Autodesk Fusion 360 part; units mm, degrees
note: some values were not read from the file. Set by a fixed rule: which sketch regions a step uses.
(part 10 of 20)
  spline S54 degree 5 poles (26.1461, -12.6495) (26.1462, -12.6495) (26.1464, -12.6496) (26.1467, -12.6497) (26.1471, -12.65) (26.1478, -12.6503) (26.1486, -12.6506) (26.1495, -12.651) (26.1504, -12.6515) (26.1515, -12.652) (26.1527, -12.6526) (26.154, -12.6531) (26.1554, -12.6538) (26.1569, -12.6544) (26.1585, -12.6551) (26.1602, -12.6559) (26.1619, -12.6567) (26.1638, -12.6575) (26.1658, -12.6583) (26.1678, -12.6592) (26.17, -12.6602) (26.1722, -12.6611) (26.1745, -12.6621) (26.1769, -12.6631) (26.1794, -12.6642) (26.182, -12.6653) (26.1847, -12.6664) (26.1874, -12.6676) (26.1903, -12.6687) (26.1932, -12.6699) (26.1962, -12.6712) (26.1993, -12.6724) (26.2024, -12.6737) (26.2057, -12.675) (26.209, -12.6764) (26.2124, -12.6778) (26.2159, -12.6791) (26.2195, -12.6806) (26.2231, -12.682) (26.2269, -12.6834) (26.2307, -12.6849) (26.2345, -12.6864) (26.2385, -12.688) (26.2425, -12.6895) (26.2466, -12.6911) (26.2508, -12.6927) (26.255, -12.6943) (26.2594, -12.6959) (26.2638, -12.6975) (26.2682, -12.6992) (26.2728, -12.7009) (26.2774, -12.7026) (26.282, -12.7043) (26.2868, -12.706) (26.2916, -12.7077) (26.2965, -12.7095) (26.3015, -12.7113) (26.3065, -12.7131) (26.3116, -12.7149) (26.3167, -12.7167) (26.322, -12.7185) (26.3273, -12.7204) (26.3326, -12.7222) (26.338, -12.7241) (26.3435, -12.726) (26.3491, -12.7279) (26.3547, -12.7298) (26.3604, -12.7317) (26.3661, -12.7336) (26.3719, -12.7356) (26.3778, -12.7375) (26.3837, -12.7395) (26.3897, -12.7414) (26.3958, -12.7434) (26.4019, -12.7454) (26.4081, -12.7474) (26.4144, -12.7494) (26.4207, -12.7514) (26.427, -12.7534) (26.4335, -12.7555) (26.4399, -12.7575) (26.4465, -12.7596) (26.4531, -12.7616) (26.4598, -12.7637) (26.4665, -12.7657) (26.4733, -12.7678) (26.4801, -12.7699) (26.487, -12.772) (26.4939, -12.774) (26.5009, -12.7761) (26.508, -12.7782) (26.5151, -12.7803) (26.5223, -12.7824) (26.5296, -12.7845) (26.5368, -12.7867) (26.5442, -12.7888) (26.5516, -12.7909) (26.559, -12.793) (26.5665, -12.7952) (26.5741, -12.7973) (26.5817, -12.7994) (26.5894, -12.8016) (26.5971, -12.8037) (26.6049, -12.8058) (26.6127, -12.808) (26.6206, -12.8101) (26.6286, -12.8123) (26.6365, -12.8144) (26.6446, -12.8166) (26.6527, -12.8187) (26.6608, -12.8208) (26.669, -12.823) (26.6773, -12.8251) (26.6856, -12.8273) (26.6939, -12.8294) (26.7023, -12.8316) (26.7108, -12.8337) (26.7193, -12.8359) (26.7278, -12.838) (26.7364, -12.8402) (26.7451, -12.8423) (26.7537, -12.8445) (26.7625, -12.8466) (26.7713, -12.8487) (26.7801, -12.8509) (26.789, -12.853) (26.798, -12.8551) (26.8069, -12.8573) (26.816, -12.8594) (26.8251, -12.8615) (26.8342, -12.8636) (26.8434, -12.8658) (26.8526, -12.8679) (26.8619, -12.87) (26.8712, -12.8721) (26.8806, -12.8742) (26.89, -12.8763) (26.8994, -12.8784) (26.9089, -12.8805) (26.9185, -12.8826) (26.9281, -12.8847) (26.9377, -12.8867) (26.9474, -12.8888) (26.9571, -12.8909) (26.9669, -12.8929) (26.9767, -12.895) (26.9866, -12.8971) (26.9965, -12.8991) (27.0064, -12.9011) (27.0164, -12.9032) (27.0265, -12.9052) (27.0365, -12.9072) (27.0467, -12.9093) (27.0568, -12.9113) (27.0671, -12.9133) (27.0773, -12.9153) (27.0876, -12.9173) (27.0979, -12.9193) (27.1083, -12.9213) (27.1188, -12.9232) (27.1292, -12.9252) (27.1397, -12.9272) (27.1503, -12.9291) (27.1609, -12.9311) (27.1715, -12.933) (27.1822, -12.9349) (27.1929, -12.9368) (27.2037, -12.9388) (27.2145, -12.9407) (27.2253, -12.9426) (27.2362, -12.9445) (27.2471, -12.9463) (27.2581, -12.9482) (27.2691, -12.9501) (27.2801, -12.9519) (27.2912, -12.9538) (27.3023, -12.9556) (27.3135, -12.9574) (27.3247, -12.9593) (27.3359, -12.9611) (27.3472, -12.9629) (27.3585, -12.9647) (27.3699, -12.9665) (27.3813, -12.9682) (27.3927, -12.97) (27.4042, -12.9718) (27.4157, -12.9735) (27.4273, -12.9752) (27.4388, -12.977) (27.4505, -12.9787) (27.4621, -12.9804) (27.4738, -12.9821) (27.4856, -12.9838) (27.4974, -12.9854) (27.5092, -12.9871) (27.521, -12.9887) (27.5329, -12.9904) (27.5449, -12.992) (27.5568, -12.9936) (27.5688, -12.9952) (27.5809, -12.9968) (27.5929, -12.9984) (27.605, -13) (27.6172, -13.0016) (27.6294, -13.0031) (27.6416, -13.0047) (27.6539, -13.0062) (27.6661, -13.0077) (27.6785, -13.0092) (27.6908, -13.0107) (27.7032, -13.0122) (27.7157, -13.0136) (27.7281, -13.0151) (27.7406, -13.0165) (27.7532, -13.018) (27.7658, -13.0194) (27.7784, -13.0208) (27.791, -13.0222) (27.8037, -13.0236) (27.8164, -13.0249) (27.8291, -13.0263) (27.8419, -13.0276) (27.8547, -13.029) (27.8676, -13.0303) (27.8805, -13.0316) (27.8934, -13.0329) (27.9063, -13.0342) (27.9193, -13.0354) (27.9323, -13.0367) (27.9454, -13.0379) (27.9585, -13.0391) (27.9716, -13.0404) (27.9848, -13.0415) (27.9979, -13.0427) (28.0112, -13.0439) (28.0244, -13.0451) (28.0377, -13.0462) (28.051, -13.0473) (28.0644, -13.0484) (28.0777, -13.0495) (28.0911, -13.0506) (28.1019, -13.0515) (28.11, -13.0521) (28.1154, -13.0525) (28.1181, -13.0527) knots 0 0 0 0 0 0 0.00416667 0.00833333 0.0125 0.01666667 0.02083333 0.025 0.02916667 0.03333333 0.0375 0.04166667 0.04583333 0.05 0.05416667 0.05833333 0.0625 0.06666667 0.07083333 0.075 0.07916667 0.08333333 0.0875 0.09166667 0.09583333 0.1 0.10416667 0.10833333 0.1125 0.11666667 0.12083333 0.125 0.12916667 0.13333333 0.1375 0.14166667 0.14583333 0.15 0.15416667 0.15833333 0.1625 0.16666667 0.17083333 0.175 0.17916667 0.18333333 0.1875 0.19166667 0.19583333 0.2 0.20416667 0.20833333 0.2125 0.21666667 0.22083333 0.225 0.22916667 0.23333333 0.2375 0.24166667 0.24583333 0.25 0.25416667 0.25833333 0.2625 0.26666667 0.27083333 0.275 0.27916667 0.28333333 0.2875 0.29166667 0.29583333 0.3 0.30416667 0.30833333 0.3125 0.31666667 0.32083333 0.325 0.32916667 0.33333333 0.3375 0.34166667 0.34583333 0.35 0.35416667 0.35833333 0.3625 0.36666667 0.37083333 0.375 0.37916667 0.38333333 0.3875 0.39166667 0.39583333 0.4 0.40416667 0.40833333 0.4125 0.41666667 0.42083333 0.425 0.42916667 0.43333333 0.4375 0.44166667 0.44583333 0.45 0.45416667 0.45833333 0.4625 0.46666667 0.47083333 0.475 0.47916667 0.48333333 0.4875 0.49166667 0.49583333 0.5 0.50416667 0.50833333 0.5125 0.51666667 0.52083333 0.525 0.52916667 0.53333333 0.5375 0.54166667 0.54583333 0.55 0.55416667 0.55833333 0.5625 0.56666667 0.57083333 0.575 0.57916667 0.58333333 0.5875 0.59166667 0.59583333 0.6 0.60416667 0.60833333 0.6125 0.61666667 0.62083333 0.625 0.62916667 0.63333333 0.6375 0.64166667 0.64583333 0.65 0.65416667 0.65833333 0.6625 0.66666667 0.67083333 0.675 0.67916667 0.68333333 0.6875 0.69166667 0.69583333 0.7 0.70416667 0.70833333 0.7125 0.71666667 0.72083333 0.725 0.72916667 0.73333333 0.7375 0.74166667 0.74583333 0.75 0.75416667 0.75833333 0.7625 0.76666667 0.77083333 0.775 0.77916667 0.78333333 0.7875 0.79166667 0.79583333 0.8 0.80416667 0.80833333 0.8125 0.81666667 0.82083333 0.825 0.82916667 0.83333333 0.8375 0.84166667 0.84583333 0.85 0.85416667 0.85833333 0.8625 0.86666667 0.87083333 0.875 0.87916667 0.88333333 0.8875 0.89166667 0.89583333 0.9 0.90416667 0.90833333 0.9125 0.91666667 0.92083333 0.925 0.92916667 0.93333333 0.9375 0.94166667 0.94583333 0.95 0.95416667 0.95833333 0.9625 0.96666667 0.97083333 0.975 0.97916667 0.98333333 0.9875 0.99166667 0.99583333 1 1 1 1 1 1
  spline S55 degree 5 poles (-25.6019, -13.7175) (-25.602, -13.7175) (-25.6022, -13.7176) (-25.6025, -13.7178) (-25.6029, -13.718) (-25.6036, -13.7184) (-25.6043, -13.7188) (-25.6052, -13.7193) (-25.6061, -13.7198) (-25.6072, -13.7204) (-25.6083, -13.721) (-25.6096, -13.7217) (-25.6109, -13.7225) (-25.6123, -13.7233) (-25.6138, -13.7242) (-25.6154, -13.7251) (-25.6171, -13.7261) (-25.6188, -13.7271) (-25.6207, -13.7282) (-25.6226, -13.7293) (-25.6246, -13.7305) (-25.6267, -13.7317) (-25.6289, -13.733) (-25.6311, -13.7344) (-25.6334, -13.7358) (-25.6358, -13.7372) (-25.6383, -13.7387) (-25.6409, -13.7403) (-25.6435, -13.7419) (-25.6462, -13.7435) (-25.6489, -13.7452) (-25.6518, -13.747) (-25.6547, -13.7488) (-25.6577, -13.7506) (-25.6607, -13.7526) (-25.6638, -13.7545) (-25.667, -13.7565) (-25.6702, -13.7586) (-25.6735, -13.7607) (-25.6769, -13.7628) (-25.6803, -13.765) (-25.6838, -13.7673) (-25.6874, -13.7696) (-25.691, -13.7719) (-25.6947, -13.7743) (-25.6984, -13.7768) (-25.7022, -13.7793) (-25.706, -13.7818) (-25.71, -13.7844) (-25.7139, -13.787) (-25.718, -13.7897) (-25.722, -13.7925) (-25.7262, -13.7952) (-25.7304, -13.7981) (-25.7346, -13.8009) (-25.7389, -13.8039) (-25.7432, -13.8068) (-25.7476, -13.8098) (-25.7521, -13.8129) (-25.7566, -13.816) (-25.7612, -13.8192) (-25.7658, -13.8224) (-25.7704, -13.8256) (-25.7751, -13.8289) (-25.7799, -13.8322) (-25.7847, -13.8356) (-25.7895, -13.839) (-25.7944, -13.8425) (-25.7993, -13.846) (-25.8043, -13.8496) (-25.8093, -13.8532) (-25.8144, -13.8568) (-25.8195, -13.8605) (-25.8247, -13.8643) (-25.8299, -13.8681) (-25.8352, -13.8719) (-25.8405, -13.8758) (-25.8458, -13.8797) (-25.8512, -13.8836) (-25.8566, -13.8876) (-25.8621, -13.8917) (-25.8676, -13.8958) (-25.8731, -13.8999) (-25.8787, -13.9041) (-25.8843, -13.9083) (-25.89, -13.9126) (-25.8957, -13.9169) (-25.9014, -13.9213) (-25.9072, -13.9257) (-25.913, -13.9301) (-25.9188, -13.9346) (-25.9247, -13.9391) (-25.9306, -13.9437) (-25.9366, -13.9483) (-25.9426, -13.9529) (-25.9486, -13.9576) (-25.9547, -13.9624) (-25.9608, -13.9672) (-25.9669, -13.972) (-25.9731, -13.9769) (-25.9793, -13.9818) (-25.9855, -13.9867) (-25.9918, -13.9917) (-25.9981, -13.9967) (-26.0044, -14.0018) (-26.0108, -14.0069) (-26.0172, -14.0121) (-26.0236, -14.0173) (-26.0301, -14.0225) (-26.0366, -14.0278) (-26.0431, -14.0332) (-26.0497, -14.0385) (-26.0563, -14.0439) (-26.0629, -14.0494) (-26.0695, -14.0549) (-26.0762, -14.0604) (-26.0829, -14.066) (-26.0896, -14.0716) (-26.0964, -14.0772) (-26.1032, -14.0829) (-26.11, -14.0887) (-26.1168, -14.0945) (-26.1237, -14.1003) (-26.1306, -14.1061) (-26.1375, -14.112) (-26.1445, -14.118) (-26.1515, -14.1239) (-26.1585, -14.13) (-26.1655, -14.136) (-26.1726, -14.1421) (-26.1796, -14.1483) (-26.1868, -14.1544) (-26.1939, -14.1607) (-26.201, -14.1669) (-26.2082, -14.1732) (-26.2154, -14.1796) (-26.2227, -14.1859) (-26.2299, -14.1924) (-26.2372, -14.1988) (-26.2445, -14.2053) (-26.2518, -14.2119) (-26.2592, -14.2184) (-26.2665, -14.225) (-26.2739, -14.2317) (-26.2813, -14.2384) (-26.2888, -14.2451) (-26.2962, -14.2519) (-26.3037, -14.2587) (-26.3112, -14.2656) (-26.3188, -14.2724) (-26.3263, -14.2794) (-26.3339, -14.2863) (-26.3414, -14.2933) (-26.3491, -14.3004) (-26.3567, -14.3075) (-26.3643, -14.3146) (-26.372, -14.3217) (-26.3797, -14.3289) (-26.3874, -14.3362) (-26.3951, -14.3435) (-26.4029, -14.3508) (-26.4106, -14.3581) (-26.4184, -14.3655) (-26.4262, -14.3729) (-26.434, -14.3804) (-26.4419, -14.3879) (-26.4497, -14.3954) (-26.4576, -14.403) (-26.4655, -14.4106) (-26.4734, -14.4183) (-26.4813, -14.426) (-26.4893, -14.4337) (-26.4972, -14.4415) (-26.5052, -14.4493) (-26.5132, -14.4571) (-26.5212, -14.465) (-26.5292, -14.4729) (-26.5373, -14.4809) (-26.5453, -14.4889) (-26.5534, -14.4969) (-26.5615, -14.505) (-26.5696, -14.5131) (-26.5777, -14.5212) (-26.5858, -14.5294) (-26.594, -14.5376) (-26.6022, -14.5459) (-26.6103, -14.5541) (-26.6185, -14.5625) (-26.6267, -14.5708) (-26.635, -14.5792) (-26.6432, -14.5877) (-26.6514, -14.5961) (-26.6597, -14.6046) (-26.668, -14.6132) (-26.6763, -14.6218) (-26.6846, -14.6304) (-26.6929, -14.639) (-26.7012, -14.6477) (-26.7096, -14.6565) (-26.7179, -14.6652) (-26.7263, -14.674) (-26.7347, -14.6829) (-26.7431, -14.6917) (-26.7515, -14.7006) (-26.7599, -14.7096) (-26.7683, -14.7186) (-26.7767, -14.7276) (-26.7852, -14.7366) (-26.7937, -14.7457) (-26.8021, -14.7549) (-26.8106, -14.764) (-26.8191, -14.7732) (-26.8276, -14.7824) (-26.8361, -14.7917) (-26.8447, -14.801) (-26.8532, -14.8104) (-26.8618, -14.8197) (-26.8703, -14.8291) (-26.8789, -14.8386) (-26.8875, -14.8481) (-26.8961, -14.8576) (-26.9047, -14.8671) (-26.9133, -14.8767) (-26.9219, -14.8863) (-26.9305, -14.896) (-26.9392, -14.9057) (-26.9478, -14.9154) (-26.9565, -14.9252) (-26.9651, -14.935) (-26.9738, -14.9448) (-26.9825, -14.9547) (-26.9912, -14.9646) (-26.9999, -14.9745) (-27.0086, -14.9845) (-27.0173, -14.9945) (-27.026, -15.0045) (-27.0347, -15.0146) (-27.0435, -15.0247) (-27.0522, -15.0349) (-27.061, -15.045) (-27.0697, -15.0553) (-27.0767, -15.0635) (-27.082, -15.0696) (-27.0855, -15.0737) (-27.0873, -15.0758) knots 0 0 0 0 0 0 0.00416667 0.00833333 0.0125 0.01666667 0.02083333 0.025 0.02916667 0.03333333 0.0375 0.04166667 0.04583333 0.05 0.05416667 0.05833333 0.0625 0.06666667 0.07083333 0.075 0.07916667 0.08333333 0.0875 0.09166667 0.09583333 0.1 0.10416667 0.10833333 0.1125 0.11666667 0.12083333 0.125 0.12916667 0.13333333 0.1375 0.14166667 0.14583333 0.15 0.15416667 0.15833333 0.1625 0.16666667 0.17083333 0.175 0.17916667 0.18333333 0.1875 0.19166667 0.19583333 0.2 0.20416667 0.20833333 0.2125 0.21666667 0.22083333 0.225 0.22916667 0.23333333 0.2375 0.24166667 0.24583333 0.25 0.25416667 0.25833333 0.2625 0.26666667 0.27083333 0.275 0.27916667 0.28333333 0.2875 0.29166667 0.29583333 0.3 0.30416667 0.30833333 0.3125 0.31666667 0.32083333 0.325 0.32916667 0.33333333 0.3375 0.34166667 0.34583333 0.35 0.35416667 0.35833333 0.3625 0.36666667 0.37083333 0.375 0.37916667 0.38333333 0.3875 0.39166667 0.39583333 0.4 0.40416667 0.40833333 0.4125 0.41666667 0.42083333 0.425 0.42916667 0.43333333 0.4375 0.44166667 0.44583333 0.45 0.45416667 0.45833333 0.4625 0.46666667 0.47083333 0.475 0.47916667 0.48333333 0.4875 0.49166667 0.49583333 0.5 0.50416667 0.50833333 0.5125 0.51666667 0.52083333 0.525 0.52916667 0.53333333 0.5375 0.54166667 0.54583333 0.55 0.55416667 0.55833333 0.5625 0.56666667 0.57083333 0.575 0.57916667 0.58333333 0.5875 0.59166667 0.59583333 0.6 0.60416667 0.60833333 0.6125 0.61666667 0.62083333 0.625 0.62916667 0.63333333 0.6375 0.64166667 0.64583333 0.65 0.65416667 0.65833333 0.6625 0.66666667 0.67083333 0.675 0.67916667 0.68333333 0.6875 0.69166667 0.69583333 0.7 0.70416667 0.70833333 0.7125 0.71666667 0.72083333 0.725 0.72916667 0.73333333 0.7375 0.74166667 0.74583333 0.75 0.75416667 0.75833333 0.7625 0.76666667 0.77083333 0.775 0.77916667 0.78333333 0.7875 0.79166667 0.79583333 0.8 0.80416667 0.80833333 0.8125 0.81666667 0.82083333 0.825 0.82916667 0.83333333 0.8375 0.84166667 0.84583333 0.85 0.85416667 0.85833333 0.8625 0.86666667 0.87083333 0.875 0.87916667 0.88333333 0.8875 0.89166667 0.89583333 0.9 0.90416667 0.90833333 0.9125 0.91666667 0.92083333 0.925 0.92916667 0.93333333 0.9375 0.94166667 0.94583333 0.95 0.95416667 0.95833333 0.9625 0.96666667 0.97083333 0.975 0.97916667 0.98333333 0.9875 0.99166667 0.99583333 1 1 1 1 1 1
  arc A56 (28.1181, -13.0527) -> (28.5147, -12.1618) centre (0, 0) ccw
  line L110 (26.8948, -10.9659) -> (26.6221, -10.8547)
  line L111 (22.1904, -18.7406) -> (22.1898, -18.7401)
  line L112 (-28.2039, -6.9368) -> (-27.918, -6.8665)
  spline S56 degree 5 poles (17.8091, 22.9448) (17.8092, 22.9448) (17.8093, 22.945) (17.8095, 22.9453) (17.8098, 22.9457) (17.8103, 22.9463) (17.8108, 22.9469) (17.8114, 22.9477) (17.812, 22.9486) (17.8127, 22.9496) (17.8135, 22.9506) (17.8144, 22.9518) (17.8153, 22.953) (17.8162, 22.9543) (17.8172, 22.9557) (17.8183, 22.9572) (17.8195, 22.9588) (17.8207, 22.9604) (17.8219, 22.9622) (17.8232, 22.964) (17.8246, 22.9659) (17.826, 22.9679) (17.8274, 22.9699) (17.8289, 22.9721) (17.8305, 22.9743) (17.8321, 22.9766) (17.8337, 22.979) (17.8354, 22.9814) (17.8372, 22.984) (17.8389, 22.9866) (17.8408, 22.9893) (17.8427, 22.992) (17.8446, 22.9948) (17.8465, 22.9978) (17.8485, 23.0007) (17.8506, 23.0038) (17.8527, 23.0069) (17.8548, 23.0101) (17.857, 23.0134) (17.8592, 23.0167) (17.8614, 23.0201) (17.8637, 23.0236) (17.866, 23.0271) (17.8683, 23.0308) (17.8707, 23.0344) (17.8731, 23.0382) (17.8756, 23.042) (17.8781, 23.0459) (17.8806, 23.0499) (17.8831, 23.0539) (17.8857, 23.058) (17.8883, 23.0621) (17.891, 23.0664) (17.8937, 23.0706) (17.8964, 23.075) (17.8991, 23.0794) (17.9019, 23.0839) (17.9047, 23.0884) (17.9075, 23.093) (17.9103, 23.0977) (17.9132, 23.1024) (17.9161, 23.1072) (17.9191, 23.1121) (17.922, 23.117) (17.925, 23.122) (17.928, 23.127) (17.931, 23.1321) (17.9341, 23.1373) (17.9372, 23.1425) (17.9403, 23.1478) (17.9434, 23.1531) (17.9466, 23.1585) (17.9497, 23.164) (17.9529, 23.1695) (17.9562, 23.1751) (17.9594, 23.1807) (17.9627, 23.1864) (17.9659, 23.1921) (17.9692, 23.1979) (17.9726, 23.2038) (17.9759, 23.2097) (17.9793, 23.2157) (17.9826, 23.2217) (17.986, 23.2278) (17.9895, 23.234) (17.9929, 23.2402) (17.9963, 23.2464) (17.9998, 23.2527) (18.0033, 23.2591) (18.0068, 23.2655) (18.0103, 23.272) (18.0139, 23.2785) (18.0174, 23.2851) (18.021, 23.2918) (18.0246, 23.2984) (18.0282, 23.3052) (18.0318, 23.312) (18.0354, 23.3188) (18.039, 23.3257) (18.0427, 23.3327) (18.0464, 23.3397) (18.0501, 23.3468) (18.0538, 23.3539) (18.0575, 23.361) (18.0612, 23.3683) (18.0649, 23.3755) (18.0687, 23.3828) (18.0724, 23.3902) (18.0762, 23.3976) (18.08, 23.4051) (18.0838, 23.4126) (18.0876, 23.4202) (18.0914, 23.4278) (18.0952, 23.4355) (18.0991, 23.4432) (18.1029, 23.451) (18.1068, 23.4588) (18.1106, 23.4666) (18.1145, 23.4746) (18.1184, 23.4825) (18.1223, 23.4905) (18.1262, 23.4986) (18.1301, 23.5067) (18.134, 23.5149) (18.1379, 23.5231) (18.1419, 23.5313) (18.1458, 23.5396) (18.1498, 23.548) (18.1537, 23.5564) (18.1577, 23.5648) (18.1617, 23.5733) (18.1657, 23.5818) (18.1696, 23.5904) (18.1736, 23.5991) (18.1776, 23.6077) (18.1816, 23.6165) (18.1857, 23.6252) (18.1897, 23.634) (18.1937, 23.6429) (18.1977, 23.6518) (18.2018, 23.6607) (18.2058, 23.6697) (18.2098, 23.6788) (18.2139, 23.6879) (18.2179, 23.697) (18.222, 23.7062) (18.226, 23.7154) (18.2301, 23.7247) (18.2342, 23.734) (18.2383, 23.7433) (18.2423, 23.7527) (18.2464, 23.7622) (18.2505, 23.7716) (18.2546, 23.7812) (18.2587, 23.7907) (18.2627, 23.8004) (18.2668, 23.81) (18.2709, 23.8197) (18.275, 23.8295) (18.2791, 23.8393) (18.2832, 23.8491) (18.2873, 23.859) (18.2914, 23.8689) (18.2955, 23.8788) (18.2996, 23.8888) (18.3038, 23.8989) (18.3079, 23.909) (18.312, 23.9191) (18.3161, 23.9292) (18.3202, 23.9395) (18.3243, 23.9497) (18.3284, 23.96) (18.3325, 23.9703) (18.3366, 23.9807) (18.3408, 23.9911) (18.3449, 24.0016) (18.349, 24.0121) (18.3531, 24.0226) (18.3572, 24.0332) (18.3613, 24.0438) (18.3654, 24.0545) (18.3695, 24.0652) (18.3736, 24.0759) (18.3777, 24.0867) (18.3818, 24.0975) (18.3859, 24.1084) (18.39, 24.1193) (18.3941, 24.1302) (18.3982, 24.1412) (18.4023, 24.1522) (18.4064, 24.1633) (18.4105, 24.1744) (18.4146, 24.1855) (18.4187, 24.1967) (18.4228, 24.2079) (18.4269, 24.2191) (18.4309, 24.2304) (18.435, 24.2417) (18.4391, 24.2531) (18.4431, 24.2645) (18.4472, 24.276) (18.4513, 24.2874) (18.4553, 24.299) (18.4594, 24.3105) (18.4634, 24.3221) (18.4675, 24.3337) (18.4715, 24.3454) (18.4756, 24.3571) (18.4796, 24.3689) (18.4836, 24.3806) (18.4877, 24.3925) (18.4917, 24.4043) (18.4957, 24.4162) (18.4997, 24.4281) (18.5037, 24.4401) (18.5077, 24.4521) (18.5117, 24.4642) (18.5157, 24.4762) (18.5197, 24.4884) (18.5237, 24.5005) (18.5277, 24.5127) (18.5316, 24.5249) (18.5356, 24.5372) (18.5395, 24.5495) (18.5435, 24.5618) (18.5475, 24.5742) (18.5514, 24.5866) (18.5553, 24.599) (18.5593, 24.6115) (18.5632, 24.624) (18.5671, 24.6365) (18.571, 24.6491) (18.5749, 24.6617) (18.5788, 24.6744) (18.5827, 24.6871) (18.5866, 24.6998) (18.5905, 24.7125) (18.5943, 24.7253) (18.5982, 24.7382) (18.6021, 24.751) (18.6059, 24.7639) (18.609, 24.7743) (18.6113, 24.782) (18.6128, 24.7872) (18.6136, 24.7898) knots 0 0 0 0 0 0 0.00416667 0.00833333 0.0125 0.01666667 0.02083333 0.025 0.02916667 0.03333333 0.0375 0.04166667 0.04583333 0.05 0.05416667 0.05833333 0.0625 0.06666667 0.07083333 0.075 0.07916667 0.08333333 0.0875 0.09166667 0.09583333 0.1 0.10416667 0.10833333 0.1125 0.11666667 0.12083333 0.125 0.12916667 0.13333333 0.1375 0.14166667 0.14583333 0.15 0.15416667 0.15833333 0.1625 0.16666667 0.17083333 0.175 0.17916667 0.18333333 0.1875 0.19166667 0.19583333 0.2 0.20416667 0.20833333 0.2125 0.21666667 0.22083333 0.225 0.22916667 0.23333333 0.2375 0.24166667 0.24583333 0.25 0.25416667 0.25833333 0.2625 0.26666667 0.27083333 0.275 0.27916667 0.28333333 0.2875 0.29166667 0.29583333 0.3 0.30416667 0.30833333 0.3125 0.31666667 0.32083333 0.325 0.32916667 0.33333333 0.3375 0.34166667 0.34583333 0.35 0.35416667 0.35833333 0.3625 0.36666667 0.37083333 0.375 0.37916667 0.38333333 0.3875 0.39166667 0.39583333 0.4 0.40416667 0.40833333 0.4125 0.41666667 0.42083333 0.425 0.42916667 0.43333333 0.4375 0.44166667 0.44583333 0.45 0.45416667 0.45833333 0.4625 0.46666667 0.47083333 0.475 0.47916667 0.48333333 0.4875 0.49166667 0.49583333 0.5 0.50416667 0.50833333 0.5125 0.51666667 0.52083333 0.525 0.52916667 0.53333333 0.5375 0.54166667 0.54583333 0.55 0.55416667 0.55833333 0.5625 0.56666667 0.57083333 0.575 0.57916667 0.58333333 0.5875 0.59166667 0.59583333 0.6 0.60416667 0.60833333 0.6125 0.61666667 0.62083333 0.625 0.62916667 0.63333333 0.6375 0.64166667 0.64583333 0.65 0.65416667 0.65833333 0.6625 0.66666667 0.67083333 0.675 0.67916667 0.68333333 0.6875 0.69166667 0.69583333 0.7 0.70416667 0.70833333 0.7125 0.71666667 0.72083333 0.725 0.72916667 0.73333333 0.7375 0.74166667 0.74583333 0.75 0.75416667 0.75833333 0.7625 0.76666667 0.77083333 0.775 0.77916667 0.78333333 0.7875 0.79166667 0.79583333 0.8 0.80416667 0.80833333 0.8125 0.81666667 0.82083333 0.825 0.82916667 0.83333333 0.8375 0.84166667 0.84583333 0.85 0.85416667 0.85833333 0.8625 0.86666667 0.87083333 0.875 0.87916667 0.88333333 0.8875 0.89166667 0.89583333 0.9 0.90416667 0.90833333 0.9125 0.91666667 0.92083333 0.925 0.92916667 0.93333333 0.9375 0.94166667 0.94583333 0.95 0.95416667 0.95833333 0.9625 0.96666667 0.97083333 0.975 0.97916667 0.98333333 0.9875 0.99166667 0.99583333 1 1 1 1 1 1
  line L113 (3.9507, 28.7745) -> (3.9508, 28.7753)
  line L114 (3.9106, 28.4828) -> (3.9507, 28.7745)
  spline S57 degree 5 poles (-26.1461, 12.6495) (-26.1462, 12.6495) (-26.1464, 12.6496) (-26.1467, 12.6497) (-26.1471, 12.65) (-26.1478, 12.6503) (-26.1486, 12.6506) (-26.1495, 12.651) (-26.1504, 12.6515) (-26.1515, 12.652) (-26.1527, 12.6526) (-26.154, 12.6531) (-26.1554, 12.6538) (-26.1569, 12.6544) (-26.1585, 12.6551) (-26.1602, 12.6559) (-26.1619, 12.6567) (-26.1638, 12.6575) (-26.1658, 12.6583) (-26.1678, 12.6592) (-26.17, 12.6602) (-26.1722, 12.6611) (-26.1745, 12.6621) (-26.1769, 12.6631) (-26.1794, 12.6642) (-26.182, 12.6653) (-26.1847, 12.6664) (-26.1874, 12.6676) (-26.1903, 12.6687) (-26.1932, 12.6699) (-26.1962, 12.6712) (-26.1993, 12.6724) (-26.2024, 12.6737) (-26.2057, 12.675) (-26.209, 12.6764) (-26.2124, 12.6778) (-26.2159, 12.6791) (-26.2195, 12.6806) (-26.2231, 12.682) (-26.2269, 12.6834) (-26.2307, 12.6849) (-26.2345, 12.6864) (-26.2385, 12.688) (-26.2425, 12.6895) (-26.2466, 12.6911) (-26.2508, 12.6927) (-26.255, 12.6943) (-26.2594, 12.6959) (-26.2638, 12.6975) (-26.2682, 12.6992) (-26.2728, 12.7009) (-26.2774, 12.7026) (-26.282, 12.7043) (-26.2868, 12.706) (-26.2916, 12.7077) (-26.2965, 12.7095) (-26.3015, 12.7113) (-26.3065, 12.7131) (-26.3116, 12.7149) (-26.3167, 12.7167) (-26.322, 12.7185) (-26.3273, 12.7204) (-26.3326, 12.7222) (-26.338, 12.7241) (-26.3435, 12.726) (-26.3491, 12.7279) (-26.3547, 12.7298) (-26.3604, 12.7317) (-26.3661, 12.7336) (-26.3719, 12.7356) (-26.3778, 12.7375) (-26.3837, 12.7395) (-26.3897, 12.7414) (-26.3958, 12.7434) (-26.4019, 12.7454) (-26.4081, 12.7474) (-26.4144, 12.7494) (-26.4207, 12.7514) (-26.427, 12.7534) (-26.4335, 12.7555) (-26.4399, 12.7575) (-26.4465, 12.7596) (-26.4531, 12.7616) (-26.4598, 12.7637) (-26.4665, 12.7657) (-26.4733, 12.7678) (-26.4801, 12.7699) (-26.487, 12.772) (-26.4939, 12.774) (-26.5009, 12.7761) (-26.508, 12.7782) (-26.5151, 12.7803) (-26.5223, 12.7824) (-26.5296, 12.7845) (-26.5368, 12.7867) (-26.5442, 12.7888) (-26.5516, 12.7909) (-26.559, 12.793) (-26.5665, 12.7952) (-26.5741, 12.7973) (-26.5817, 12.7994) (-26.5894, 12.8016) (-26.5971, 12.8037) (-26.6049, 12.8058) (-26.6127, 12.808) (-26.6206, 12.8101) (-26.6286, 12.8123) (-26.6365, 12.8144) (-26.6446, 12.8166) (-26.6527, 12.8187) (-26.6608, 12.8208) (-26.669, 12.823) (-26.6773, 12.8251) (-26.6856, 12.8273) (-26.6939, 12.8294) (-26.7023, 12.8316) (-26.7108, 12.8337) (-26.7193, 12.8359) (-26.7278, 12.838) (-26.7364, 12.8402) (-26.7451, 12.8423) (-26.7537, 12.8445) (-26.7625, 12.8466) (-26.7713, 12.8487) (-26.7801, 12.8509) (-26.789, 12.853) (-26.798, 12.8551) (-26.8069, 12.8573) (-26.816, 12.8594) (-26.8251, 12.8615) (-26.8342, 12.8636) (-26.8434, 12.8658) (-26.8526, 12.8679) (-26.8619, 12.87) (-26.8712, 12.8721) (-26.8806, 12.8742) (-26.89, 12.8763) (-26.8994, 12.8784) (-26.9089, 12.8805) (-26.9185, 12.8826) (-26.9281, 12.8847) (-26.9377, 12.8867) (-26.9474, 12.8888) (-26.9571, 12.8909) (-26.9669, 12.8929) (-26.9767, 12.895) (-26.9866, 12.8971) (-26.9965, 12.8991) (-27.0064, 12.9011) (-27.0164, 12.9032) (-27.0265, 12.9052) (-27.0365, 12.9072) (-27.0467, 12.9093) (-27.0568, 12.9113) (-27.0671, 12.9133) (-27.0773, 12.9153) (-27.0876, 12.9173) (-27.0979, 12.9193) (-27.1083, 12.9213) (-27.1188, 12.9232) (-27.1292, 12.9252) (-27.1397, 12.9272) (-27.1503, 12.9291) (-27.1609, 12.9311) (-27.1715, 12.933) (-27.1822, 12.9349) (-27.1929, 12.9368) (-27.2037, 12.9388) (-27.2145, 12.9407) (-27.2253, 12.9426) (-27.2362, 12.9445) (-27.2471, 12.9463) (-27.2581, 12.9482) (-27.2691, 12.9501) (-27.2801, 12.9519) (-27.2912, 12.9538) (-27.3023, 12.9556) (-27.3135, 12.9574) (-27.3247, 12.9593) (-27.3359, 12.9611) (-27.3472, 12.9629) (-27.3585, 12.9647) (-27.3699, 12.9665) (-27.3813, 12.9682) (-27.3927, 12.97) (-27.4042, 12.9718) (-27.4157, 12.9735) (-27.4273, 12.9752) (-27.4388, 12.977) (-27.4505, 12.9787) (-27.4621, 12.9804) (-27.4738, 12.9821) (-27.4856, 12.9838) (-27.4974, 12.9854) (-27.5092, 12.9871) (-27.521, 12.9887) (-27.5329, 12.9904) (-27.5449, 12.992) (-27.5568, 12.9936) (-27.5688, 12.9952) (-27.5809, 12.9968) (-27.5929, 12.9984) (-27.605, 13) (-27.6172, 13.0016) (-27.6294, 13.0031) (-27.6416, 13.0047) (-27.6539, 13.0062) (-27.6661, 13.0077) (-27.6785, 13.0092) (-27.6908, 13.0107) (-27.7032, 13.0122) (-27.7157, 13.0136) (-27.7281, 13.0151) (-27.7406, 13.0165) (-27.7532, 13.018) (-27.7658, 13.0194) (-27.7784, 13.0208) (-27.791, 13.0222) (-27.8037, 13.0236) (-27.8164, 13.0249) (-27.8291, 13.0263) (-27.8419, 13.0276) (-27.8547, 13.029) (-27.8676, 13.0303) (-27.8805, 13.0316) (-27.8934, 13.0329) (-27.9063, 13.0342) (-27.9193, 13.0354) (-27.9323, 13.0367) (-27.9454, 13.0379) (-27.9585, 13.0391) (-27.9716, 13.0404) (-27.9848, 13.0415) (-27.9979, 13.0427) (-28.0112, 13.0439) (-28.0244, 13.0451) (-28.0377, 13.0462) (-28.051, 13.0473) (-28.0644, 13.0484) (-28.0777, 13.0495) (-28.0911, 13.0506) (-28.1019, 13.0515) (-28.11, 13.0521) (-28.1154, 13.0525) (-28.1181, 13.0527) knots 0 0 0 0 0 0 0.00416667 0.00833333 0.0125 0.01666667 0.02083333 0.025 0.02916667 0.03333333 0.0375 0.04166667 0.04583333 0.05 0.05416667 0.05833333 0.0625 0.06666667 0.07083333 0.075 0.07916667 0.08333333 0.0875 0.09166667 0.09583333 0.1 0.10416667 0.10833333 0.1125 0.11666667 0.12083333 0.125 0.12916667 0.13333333 0.1375 0.14166667 0.14583333 0.15 0.15416667 0.15833333 0.1625 0.16666667 0.17083333 0.175 0.17916667 0.18333333 0.1875 0.19166667 0.19583333 0.2 0.20416667 0.20833333 0.2125 0.21666667 0.22083333 0.225 0.22916667 0.23333333 0.2375 0.24166667 0.24583333 0.25 0.25416667 0.25833333 0.2625 0.26666667 0.27083333 0.275 0.27916667 0.28333333 0.2875 0.29166667 0.29583333 0.3 0.30416667 0.30833333 0.3125 0.31666667 0.32083333 0.325 0.32916667 0.33333333 0.3375 0.34166667 0.34583333 0.35 0.35416667 0.35833333 0.3625 0.36666667 0.37083333 0.375 0.37916667 0.38333333 0.3875 0.39166667 0.39583333 0.4 0.40416667 0.40833333 0.4125 0.41666667 0.42083333 0.425 0.42916667 0.43333333 0.4375 0.44166667 0.44583333 0.45 0.45416667 0.45833333 0.4625 0.46666667 0.47083333 0.475 0.47916667 0.48333333 0.4875 0.49166667 0.49583333 0.5 0.50416667 0.50833333 0.5125 0.51666667 0.52083333 0.525 0.52916667 0.53333333 0.5375 0.54166667 0.54583333 0.55 0.55416667 0.55833333 0.5625 0.56666667 0.57083333 0.575 0.57916667 0.58333333 0.5875 0.59166667 0.59583333 0.6 0.60416667 0.60833333 0.6125 0.61666667 0.62083333 0.625 0.62916667 0.63333333 0.6375 0.64166667 0.64583333 0.65 0.65416667 0.65833333 0.6625 0.66666667 0.67083333 0.675 0.67916667 0.68333333 0.6875 0.69166667 0.69583333 0.7 0.70416667 0.70833333 0.7125 0.71666667 0.72083333 0.725 0.72916667 0.73333333 0.7375 0.74166667 0.74583333 0.75 0.75416667 0.75833333 0.7625 0.76666667 0.77083333 0.775 0.77916667 0.78333333 0.7875 0.79166667 0.79583333 0.8 0.80416667 0.80833333 0.8125 0.81666667 0.82083333 0.825 0.82916667 0.83333333 0.8375 0.84166667 0.84583333 0.85 0.85416667 0.85833333 0.8625 0.86666667 0.87083333 0.875 0.87916667 0.88333333 0.8875 0.89166667 0.89583333 0.9 0.90416667 0.90833333 0.9125 0.91666667 0.92083333 0.925 0.92916667 0.93333333 0.9375 0.94166667 0.94583333 0.95 0.95416667 0.95833333 0.9625 0.96666667 0.97083333 0.975 0.97916667 0.98333333 0.9875 0.99166667 0.99583333 1 1 1 1 1 1
  arc A57 (-28.1181, 13.0527) -> (-28.5147, 12.1618) centre (0, 0) ccw
  spline S58 degree 5 poles (-28.5147, 12.1618) (-28.5128, 12.16) (-28.5089, 12.1562) (-28.503, 12.1506) (-28.4951, 12.1432) (-28.4854, 12.134) (-28.4756, 12.1248) (-28.4658, 12.1156) (-28.4561, 12.1065) (-28.4464, 12.0973) (-28.4366, 12.0883) (-28.4269, 12.0792) (-28.4172, 12.0702) (-28.4075, 12.0613) (-28.3978, 12.0523) (-28.3882, 12.0434) (-28.3785, 12.0345) (-28.3689, 12.0257) (-28.3593, 12.0169) (-28.3496, 12.0081) (-28.34, 11.9994) (-28.3305, 11.9907) (-28.3209, 11.982) (-28.3113, 11.9734) (-28.3018, 11.9648) (-28.2922, 11.9562) (-28.2827, 11.9477) (-28.2732, 11.9392) (-28.2637, 11.9307) (-28.2542, 11.9223) (-28.2447, 11.9139) (-28.2353, 11.9055) (-28.2259, 11.8972) (-28.2164, 11.8889) (-28.207, 11.8807) (-28.1976, 11.8724) (-28.1882, 11.8643) (-28.1789, 11.8561) (-28.1695, 11.848) (-28.1602, 11.8399) (-28.1509, 11.8318) (-28.1416, 11.8238) (-28.1323, 11.8158) (-28.123, 11.8079) (-28.1137, 11.8) (-28.1045, 11.7921) (-28.0953, 11.7843) (-28.0861, 11.7765) (-28.0769, 11.7687) (-28.0677, 11.7609) (-28.0585, 11.7532) (-28.0494, 11.7456) (-28.0403, 11.7379) (-28.0312, 11.7303) (-28.0221, 11.7228) (-28.013, 11.7153) (-28.0039, 11.7078) (-27.9949, 11.7003) (-27.9859, 11.6929) (-27.9769, 11.6855) (-27.9679, 11.6781) (-27.9589, 11.6708) (-27.95, 11.6635) (-27.9411, 11.6563) (-27.9322, 11.6491) (-27.9233, 11.6419) (-27.9144, 11.6348) (-27.9055, 11.6276) (-27.8967, 11.6206) (-27.8879, 11.6135) (-27.8791, 11.6065) (-27.8704, 11.5996) (-27.8616, 11.5927) (-27.8529, 11.5858) (-27.8442, 11.5789) (-27.8355, 11.5721) (-27.8268, 11.5653) (-27.8182, 11.5585) (-27.8096, 11.5518) (-27.801, 11.5452) (-27.7924, 11.5385) (-27.7838, 11.5319) (-27.7753, 11.5253) (-27.7668, 11.5188) (-27.7583, 11.5123) (-27.7498, 11.5058) (-27.7414, 11.4994) (-27.733, 11.493) (-27.7246, 11.4867) (-27.7162, 11.4803) (-27.7078, 11.4741) (-27.6995, 11.4678) (-27.6912, 11.4616) (-27.6829, 11.4554) (-27.6747, 11.4493) (-27.6665, 11.4432) (-27.6582, 11.4371) (-27.6501, 11.4311) (-27.6419, 11.4251) (-27.6338, 11.4192) (-27.6257, 11.4132) (-27.6176, 11.4074) (-27.6096, 11.4015) (-27.6015, 11.3957) (-27.5936, 11.3899) (-27.5856, 11.3842) (-27.5776, 11.3785) (-27.5697, 11.3728) (-27.5618, 11.3672) (-27.554, 11.3616) (-27.5462, 11.3561) (-27.5384, 11.3506) (-27.5306, 11.3451) (-27.5228, 11.3396) (-27.5151, 11.3342) (-27.5074, 11.3289) (-27.4998, 11.3235) (-27.4922, 11.3183) (-27.4846, 11.313) (-27.477, 11.3078) (-27.4695, 11.3026) (-27.462, 11.2975) (-27.4545, 11.2924) (-27.447, 11.2873) (-27.4396, 11.2823) (-27.4323, 11.2773) (-27.4249, 11.2723) (-27.4176, 11.2674) (-27.4103, 11.2625) (-27.4031, 11.2577) (-27.3958, 11.2529) (-27.3887, 11.2481) (-27.3815, 11.2434) (-27.3744, 11.2387) (-27.3673, 11.234) (-27.3603, 11.2294) (-27.3533, 11.2248) (-27.3463, 11.2203) (-27.3393, 11.2158) (-27.3324, 11.2113) (-27.3256, 11.2069) (-27.3187, 11.2025) (-27.3119, 11.1982) (-27.3052, 11.1939) (-27.2985, 11.1896) (-27.2918, 11.1854) (-27.2851, 11.1812) (-27.2785, 11.177) (-27.272, 11.1729) (-27.2654, 11.1688) (-27.259, 11.1648) (-27.2525, 11.1608) (-27.2461, 11.1568) (-27.2397, 11.1529) (-27.2334, 11.149) (-27.2271, 11.1451) (-27.2209, 11.1413) (-27.2147, 11.1376) (-27.2085, 11.1338) (-27.2024, 11.1301) (-27.1963, 11.1265) (-27.1903, 11.1229) (-27.1843, 11.1193) (-27.1784, 11.1158) (-27.1725, 11.1123) (-27.1666, 11.1088) (-27.1608, 11.1054) (-27.155, 11.102) (-27.1493, 11.0987) (-27.1436, 11.0954) (-27.138, 11.0921) (-27.1324, 11.0889) (-27.1269, 11.0857) (-27.1214, 11.0826) (-27.116, 11.0795) (-27.1106, 11.0764) (-27.1053, 11.0734) (-27.1, 11.0704) (-27.0948, 11.0675) (-27.0896, 11.0646) (-27.0845, 11.0617) (-27.0794, 11.0589) (-27.0744, 11.0561) (-27.0694, 11.0534) (-27.0645, 11.0507) (-27.0597, 11.048) (-27.0549, 11.0454) (-27.0501, 11.0428) (-27.0454, 11.0403) (-27.0408, 11.0378) (-27.0362, 11.0353) (-27.0317, 11.0329) (-27.0272, 11.0306) (-27.0228, 11.0282) (-27.0185, 11.0259) (-27.0142, 11.0237) (-27.01, 11.0215) (-27.0058, 11.0193) (-27.0017, 11.0172) (-26.9977, 11.0151) (-26.9937, 11.0131) (-26.9898, 11.0111) (-26.986, 11.0091) (-26.9822, 11.0072) (-26.9785, 11.0053) (-26.9748, 11.0035) (-26.9713, 11.0017) (-26.9678, 10.9999) (-26.9643, 10.9982) (-26.961, 10.9966) (-26.9577, 10.9949) (-26.9544, 10.9934) (-26.9513, 10.9918) (-26.9482, 10.9903) (-26.9452, 10.9889) (-26.9423, 10.9875) (-26.9394, 10.9861) (-26.9366, 10.9848) (-26.9339, 10.9835) (-26.9313, 10.9823) (-26.9288, 10.9811) (-26.9263, 10.9799) (-26.924, 10.9788) (-26.9217, 10.9778) (-26.9195, 10.9768) (-26.9173, 10.9758) (-26.9153, 10.9749) (-26.9134, 10.974) (-26.9115, 10.9731) (-26.9097, 10.9724) (-26.908, 10.9716) (-26.9065, 10.9709) (-26.905, 10.9702) (-26.9036, 10.9696) (-26.9023, 10.9691) (-26.9011, 10.9685) (-26.9, 10.9681) (-26.899, 10.9676) (-26.8981, 10.9672) (-26.8973, 10.9669) (-26.8966, 10.9666) (-26.8961, 10.9664) (-26.8958, 10.9663) (-26.8956, 10.9662) (-26.8955, 10.9662) knots -1 -1 -1 -1 -1 -1 -0.99583333 -0.99166667 -0.9875 -0.98333333 -0.97916667 -0.975 -0.97083333 -0.96666667 -0.9625 -0.95833333 -0.95416667 -0.95 -0.94583333 -0.94166667 -0.9375 -0.93333333 -0.92916667 -0.925 -0.92083333 -0.91666667 -0.9125 -0.90833333 -0.90416667 -0.9 -0.89583333 -0.89166667 -0.8875 -0.88333333 -0.87916667 -0.875 -0.87083333 -0.86666667 -0.8625 -0.85833333 -0.85416667 -0.85 -0.84583333 -0.84166667 -0.8375 -0.83333333 -0.82916667 -0.825 -0.82083333 -0.81666667 -0.8125 -0.80833333 -0.80416667 -0.8 -0.79583333 -0.79166667 -0.7875 -0.78333333 -0.77916667 -0.775 -0.77083333 -0.76666667 -0.7625 -0.75833333 -0.75416667 -0.75 -0.74583333 -0.74166667 -0.7375 -0.73333333 -0.72916667 -0.725 -0.72083333 -0.71666667 -0.7125 -0.70833333 -0.70416667 -0.7 -0.69583333 -0.69166667 -0.6875 -0.68333333 -0.67916667 -0.675 -0.67083333 -0.66666667 -0.6625 -0.65833333 -0.65416667 -0.65 -0.64583333 -0.64166667 -0.6375 -0.63333333 -0.62916667 -0.625 -0.62083333 -0.61666667 -0.6125 -0.60833333 -0.60416667 -0.6 -0.59583333 -0.59166667 -0.5875 -0.58333333 -0.57916667 -0.575 -0.57083333 -0.56666667 -0.5625 -0.55833333 -0.55416667 -0.55 -0.54583333 -0.54166667 -0.5375 -0.53333333 -0.52916667 -0.525 -0.52083333 -0.51666667 -0.5125 -0.50833333 -0.50416667 -0.5 -0.49583333 -0.49166667 -0.4875 -0.48333333 -0.47916667 -0.475 -0.47083333 -0.46666667 -0.4625 -0.45833333 -0.45416667 -0.45 -0.44583333 -0.44166667 -0.4375 -0.43333333 -0.42916667 -0.425 -0.42083333 -0.41666667 -0.4125 -0.40833333 -0.40416667 -0.4 -0.39583333 -0.39166667 -0.3875 -0.38333333 -0.37916667 -0.375 -0.37083333 -0.36666667 -0.3625 -0.35833333 -0.35416667 -0.35 -0.34583333 -0.34166667 -0.3375 -0.33333333 -0.32916667 -0.325 -0.32083333 -0.31666667 -0.3125 -0.30833333 -0.30416667 -0.3 -0.29583333 -0.29166667 -0.2875 -0.28333333 -0.27916667 -0.275 -0.27083333 -0.26666667 -0.2625 -0.25833333 -0.25416667 -0.25 -0.24583333 -0.24166667 -0.2375 -0.23333333 -0.22916667 -0.225 -0.22083333 -0.21666667 -0.2125 -0.20833333 -0.20416667 -0.2 -0.19583333 -0.19166667 -0.1875 -0.18333333 -0.17916667 -0.175 -0.17083333 -0.16666667 -0.1625 -0.15833333 -0.15416667 -0.15 -0.14583333 -0.14166667 -0.1375 -0.13333333 -0.12916667 -0.125 -0.12083333 -0.11666667 -0.1125 -0.10833333 -0.10416667 -0.1 -0.09583333 -0.09166667 -0.0875 -0.08333333 -0.07916667 -0.075 -0.07083333 -0.06666667 -0.0625 -0.05833333 -0.05416667 -0.05 -0.04583333 -0.04166667 -0.0375 -0.03333333 -0.02916667 -0.025 -0.02083333 -0.01666667 -0.0125 -0.00833333 -0.00416667 0 0 0 0 0 0
  spline S59 degree 5 poles (-0.4876, 30.9962) (-0.4885, 30.9936) (-0.4903, 30.9885) (-0.493, 30.9809) (-0.4966, 30.9707) (-0.5011, 30.958) (-0.5055, 30.9453) (-0.5099, 30.9327) (-0.5143, 30.9201) (-0.5187, 30.9075) (-0.523, 30.8949) (-0.5273, 30.8823) (-0.5316, 30.8698) (-0.5359, 30.8573) (-0.5401, 30.8448) (-0.5443, 30.8324) (-0.5485, 30.82) (-0.5526, 30.8076) (-0.5568, 30.7952) (-0.5609, 30.7828) (-0.5649, 30.7705) (-0.569, 30.7582) (-0.573, 30.7459) (-0.577, 30.7337) (-0.581, 30.7215) (-0.5849, 30.7093) (-0.5889, 30.6971) (-0.5927, 30.685) (-0.5966, 30.6728) (-0.6005, 30.6607) (-0.6043, 30.6487) (-0.6081, 30.6366) (-0.6118, 30.6246) (-0.6156, 30.6126) (-0.6193, 30.6007) (-0.623, 30.5888) (-0.6267, 30.5769) (-0.6303, 30.565) (-0.6339, 30.5531) (-0.6375, 30.5413) (-0.6411, 30.5295) (-0.6446, 30.5178) (-0.6481, 30.506) (-0.6516, 30.4943) (-0.6551, 30.4827) (-0.6585, 30.471) (-0.6619, 30.4594) (-0.6653, 30.4478) (-0.6687, 30.4362) (-0.672, 30.4247) (-0.6753, 30.4132) (-0.6786, 30.4017) (-0.6819, 30.3903) (-0.6851, 30.3789) (-0.6883, 30.3675) (-0.6915, 30.3562) (-0.6947, 30.3448) (-0.6978, 30.3336) (-0.7009, 30.3223) (-0.704, 30.3111) (-0.7071, 30.2999) (-0.7101, 30.2887) (-0.7131, 30.2776) (-0.7161, 30.2665) (-0.7191, 30.2554) (-0.722, 30.2444) (-0.7249, 30.2334) (-0.7278, 30.2224) (-0.7307, 30.2114) (-0.7335, 30.2005) (-0.7364, 30.1897) (-0.7391, 30.1788) (-0.7419, 30.168) (-0.7447, 30.1572) (-0.7474, 30.1465) (-0.7501, 30.1358) (-0.7528, 30.1251) (-0.7554, 30.1145) (-0.758, 30.1038) (-0.7606, 30.0933) (-0.7632, 30.0827) (-0.7658, 30.0722) (-0.7683, 30.0618) (-0.7708, 30.0513) (-0.7733, 30.0409) (-0.7758, 30.0306) (-0.7782, 30.0202) (-0.7806, 30.0099) (-0.783, 29.9997) (-0.7854, 29.9895) (-0.7877, 29.9793) (-0.79, 29.9691) (-0.7923, 29.959) (-0.7946, 29.949) (-0.7969, 29.9389) (-0.7991, 29.9289) (-0.8013, 29.919) (-0.8035, 29.909) (-0.8056, 29.8992) (-0.8078, 29.8893) (-0.8099, 29.8795) (-0.812, 29.8697) (-0.814, 29.86) (-0.8161, 29.8503) (-0.8181, 29.8407) (-0.8201, 29.8311) (-0.8221, 29.8215) (-0.824, 29.812) (-0.8259, 29.8025) (-0.8279, 29.793) (-0.8297, 29.7836) (-0.8316, 29.7742) (-0.8334, 29.7649) (-0.8353, 29.7556) (-0.8371, 29.7464) (-0.8388, 29.7372) (-0.8406, 29.728) (-0.8423, 29.7189) (-0.844, 29.7098) (-0.8457, 29.7008) (-0.8474, 29.6918) (-0.849, 29.6828) (-0.8507, 29.6739) (-0.8523, 29.6651) (-0.8538, 29.6563) (-0.8554, 29.6475) (-0.8569, 29.6388) (-0.8585, 29.6301) (-0.86, 29.6214) (-0.8614, 29.6128) (-0.8629, 29.6043) (-0.8643, 29.5958) (-0.8657, 29.5873) (-0.8671, 29.5789) (-0.8685, 29.5706) (-0.8698, 29.5623) (-0.8712, 29.554) (-0.8725, 29.5458) (-0.8738, 29.5376) (-0.875, 29.5295) (-0.8763, 29.5214) (-0.8775, 29.5134) (-0.8787, 29.5054) (-0.8799, 29.4975) (-0.8811, 29.4896) (-0.8822, 29.4818) (-0.8834, 29.474) (-0.8845, 29.4663) (-0.8856, 29.4586) (-0.8866, 29.451) (-0.8877, 29.4434) (-0.8887, 29.4359) (-0.8897, 29.4284) (-0.8907, 29.421) (-0.8917, 29.4137) (-0.8927, 29.4063) (-0.8936, 29.3991) (-0.8945, 29.3919) (-0.8954, 29.3847) (-0.8963, 29.3777) (-0.8972, 29.3706) (-0.898, 29.3636) (-0.8989, 29.3567) (-0.8997, 29.3498) (-0.9005, 29.343) (-0.9012, 29.3363) (-0.902, 29.3296) (-0.9027, 29.323) (-0.9035, 29.3164) (-0.9042, 29.3099) (-0.9049, 29.3034) (-0.9055, 29.297) (-0.9062, 29.2906) (-0.9068, 29.2844) (-0.9075, 29.2781) (-0.9081, 29.272) (-0.9087, 29.2659) (-0.9092, 29.2599) (-0.9098, 29.2539) (-0.9103, 29.248) (-0.9109, 29.2421) (-0.9114, 29.2363) (-0.9119, 29.2306) (-0.9124, 29.225) (-0.9128, 29.2194) (-0.9133, 29.2139) (-0.9137, 29.2084) (-0.9141, 29.203) (-0.9146, 29.1977) (-0.915, 29.1925) (-0.9153, 29.1873) (-0.9157, 29.1822) (-0.9161, 29.1771) (-0.9164, 29.1722) (-0.9167, 29.1673) (-0.917, 29.1624) (-0.9173, 29.1577) (-0.9176, 29.153) (-0.9179, 29.1484) (-0.9182, 29.1439) (-0.9184, 29.1394) (-0.9186, 29.135) (-0.9189, 29.1307) (-0.9191, 29.1265) (-0.9193, 29.1223) (-0.9195, 29.1183) (-0.9197, 29.1143) (-0.9198, 29.1103) (-0.92, 29.1065) (-0.9201, 29.1028) (-0.9203, 29.0991) (-0.9204, 29.0955) (-0.9205, 29.092) (-0.9206, 29.0886) (-0.9208, 29.0852) (-0.9208, 29.082) (-0.9209, 29.0788) (-0.921, 29.0758) (-0.9211, 29.0728) (-0.9211, 29.0699) (-0.9212, 29.0671) (-0.9212, 29.0644) (-0.9213, 29.0618) (-0.9213, 29.0592) (-0.9214, 29.0568) (-0.9214, 29.0545) (-0.9214, 29.0522) (-0.9214, 29.0501) (-0.9214, 29.0481) (-0.9214, 29.0461) (-0.9214, 29.0443) (-0.9214, 29.0425) (-0.9214, 29.0409) (-0.9214, 29.0394) (-0.9214, 29.038) (-0.9214, 29.0367) (-0.9214, 29.0355) (-0.9214, 29.0344) (-0.9213, 29.0334) (-0.9213, 29.0325) (-0.9213, 29.0318) (-0.9213, 29.0313) (-0.9213, 29.0309) (-0.9213, 29.0307) (-0.9213, 29.0307) knots -1 -1 -1 -1 -1 -1 -0.99583333 -0.99166667 -0.9875 -0.98333333 -0.97916667 -0.975 -0.97083333 -0.96666667 -0.9625 -0.95833333 -0.95416667 -0.95 -0.94583333 -0.94166667 -0.9375 -0.93333333 -0.92916667 -0.925 -0.92083333 -0.91666667 -0.9125 -0.90833333 -0.90416667 -0.9 -0.89583333 -0.89166667 -0.8875 -0.88333333 -0.87916667 -0.875 -0.87083333 -0.86666667 -0.8625 -0.85833333 -0.85416667 -0.85 -0.84583333 -0.84166667 -0.8375 -0.83333333 -0.82916667 -0.825 -0.82083333 -0.81666667 -0.8125 -0.80833333 -0.80416667 -0.8 -0.79583333 -0.79166667 -0.7875 -0.78333333 -0.77916667 -0.775 -0.77083333 -0.76666667 -0.7625 -0.75833333 -0.75416667 -0.75 -0.74583333 -0.74166667 -0.7375 -0.73333333 -0.72916667 -0.725 -0.72083333 -0.71666667 -0.7125 -0.70833333 -0.70416667 -0.7 -0.69583333 -0.69166667 -0.6875 -0.68333333 -0.67916667 -0.675 -0.67083333 -0.66666667 -0.6625 -0.65833333 -0.65416667 -0.65 -0.64583333 -0.64166667 -0.6375 -0.63333333 -0.62916667 -0.625 -0.62083333 -0.61666667 -0.6125 -0.60833333 -0.60416667 -0.6 -0.59583333 -0.59166667 -0.5875 -0.58333333 -0.57916667 -0.575 -0.57083333 -0.56666667 -0.5625 -0.55833333 -0.55416667 -0.55 -0.54583333 -0.54166667 -0.5375 -0.53333333 -0.52916667 -0.525 -0.52083333 -0.51666667 -0.5125 -0.50833333 -0.50416667 -0.5 -0.49583333 -0.49166667 -0.4875 -0.48333333 -0.47916667 -0.475 -0.47083333 -0.46666667 -0.4625 -0.45833333 -0.45416667 -0.45 -0.44583333 -0.44166667 -0.4375 -0.43333333 -0.42916667 -0.425 -0.42083333 -0.41666667 -0.4125 -0.40833333 -0.40416667 -0.4 -0.39583333 -0.39166667 -0.3875 -0.38333333 -0.37916667 -0.375 -0.37083333 -0.36666667 -0.3625 -0.35833333 -0.35416667 -0.35 -0.34583333 -0.34166667 -0.3375 -0.33333333 -0.32916667 -0.325 -0.32083333 -0.31666667 -0.3125 -0.30833333 -0.30416667 -0.3 -0.29583333 -0.29166667 -0.2875 -0.28333333 -0.27916667 -0.275 -0.27083333 -0.26666667 -0.2625 -0.25833333 -0.25416667 -0.25 -0.24583333 -0.24166667 -0.2375 -0.23333333 -0.22916667 -0.225 -0.22083333 -0.21666667 -0.2125 -0.20833333 -0.20416667 -0.2 -0.19583333 -0.19166667 -0.1875 -0.18333333 -0.17916667 -0.175 -0.17083333 -0.16666667 -0.1625 -0.15833333 -0.15416667 -0.15 -0.14583333 -0.14166667 -0.1375 -0.13333333 -0.12916667 -0.125 -0.12083333 -0.11666667 -0.1125 -0.10833333 -0.10416667 -0.1 -0.09583333 -0.09166667 -0.0875 -0.08333333 -0.07916667 -0.075 -0.07083333 -0.06666667 -0.0625 -0.05833333 -0.05416667 -0.05 -0.04583333 -0.04166667 -0.0375 -0.03333333 -0.02916667 -0.025 -0.02083333 -0.01666667 -0.0125 -0.00833333 -0.00416667 0 0 0 0 0 0
  arc A58 (-17.6281, 22.7115) -> (-18.5501, 21.9649) centre (0, 0) ccw
  arc A59 (-2.755, 30.8773) -> (-3.7249, 30.7754) centre (0, 0) ccw
  line L115 (27.3251, 9.8472) -> (27.3243, 9.8469)
  line L116 (26.6221, 10.8547) -> (26.8948, 10.9659)
  line L117 (-3.9508, 28.7753) -> (-3.9507, 28.7745)
  arc A60 (-6.9214, -30.2174) -> (-5.9675, -30.4202) centre (0, 0) ccw
  line L118 (-3.9507, 28.7745) -> (-3.9106, 28.4828)
  line L119 (-2.1182, 28.9671) -> (-2.1183, 28.9679)